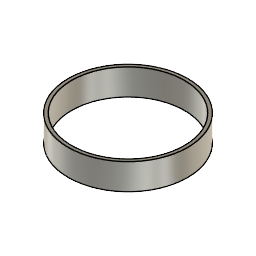
Φ457.2×12.7 (Autodesk Fusion 360 design; units mm, degrees)
Autodesk Fusion 360 part; units mm, degrees
sketch "スケッチ1" plane through (0, 0, 0) normal (0, 0, 1) x (1, 0, 0)
  circle A0 centre (0, 0) radius 228.6
  circle A1 centre (0, 0) radius 215.9
  dimension "d1" = 457.2
  dimension "d2" = -12.7
  constraint coincident A0.centre A1.centre
  measures "d1" diameter of A0
extrude "押し出し1" add sketch "スケッチ1" along normal blind 100
